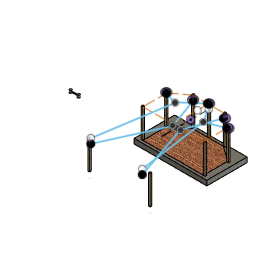
Mic Placements v4 (Autodesk Fusion 360 design; units mm, degrees)
Autodesk Fusion 360 part; units mm, degrees
sketch "Sketch1" plane through (0, 0, 0) normal (0, 1, 0) x (1, 0, 0)
  line L0 (0, 1104.9) -> (0, -342.9) construction
  line L1 (-1905, 1104.9) -> (1905, 1104.9) construction
  line L2 (-1905, -1104.9) -> (1905, -1104.9)
  line L3 (1905, -1104.9) -> (-1905, 1104.9) construction
  line L4 (-1905, -1104.9) -> (-1905, 1104.9) construction
  line L5 (0, -342.9) -> (0, 419.1) construction
  line L6 (0, 1104.9) -> (0, -342.9) construction
  line L7 (-1905, 419.1) -> (-952.5, 1104.9)
  line L8 (-1905, -342.9) -> (-1905, 1104.9) construction
  line L9 (-1905, 419.1) -> (-1905, -1104.9)
  line L10 (1905, 1104.9) -> (1905, -1104.9) construction
  line L11 (-1905, 1104.9) -> (0, 1104.9) construction
  line L12 (1905, -342.9) -> (1905, 1104.9) construction
  line L13 (1905, -342.9) -> (1905, 419.1) construction
  line L14 (0, -342.9) -> (1905, -342.9) construction
  line L15 (1905, 1104.9) -> (0, 1104.9) construction
  line L16 (1905, 419.1) -> (952.5, 1104.9) construction
  line L17 (-952.5, 1104.9) -> (952.5, 1104.9)
  line L18 (0, 1104.9) -> (0, -342.9) construction
  line L19 (1905, 419.1) -> (-1905, 419.1)
  line L20 (1905, -1104.9) -> (1905, 419.1)
  line L21 (-1905, -1104.9) -> (1905, 1104.9) construction
  line L22 (1905, -1104.9) -> (-1905, -1104.9) construction
  line L23 (0, -342.9) -> (-1905, -342.9) construction
  line L24 (1905, 419.1) -> (952.5, 1104.9)
  line L25 (1905, 419.1) -> (0, 419.1) construction
  line L26 (50.7492, 1206.3984) -> (50.7492, 1104.9)
  line L27 (952.5, 1104.9) -> (-952.5, 1104.9)
  line L28 (-1905, -1104.9) -> (1905, -1104.9)
  line L29 (-1905, -1104.9) -> (-2006.4984, -1104.9)
  line L30 (-2006.4984, 368.3508) -> (-2006.4984, 469.8492)
  line L31 (-1905, -1003.4016) -> (-1905, -1104.9)
  line L32 (952.5, 1104.9) -> (1054.1, 1104.9)
  line L33 (1054.1, 1206.5) -> (952.5, 1206.5)
  line L34 (1905, 419.1) -> (952.5, 1104.9)
  line L35 (0, 1104.9) -> (0, -1104.9) construction
  line L36 (1905, -1104.9) -> (2006.4984, -1104.9)
  line L37 (-1905, 368.3508) -> (-2006.4984, 469.8492) construction
  line L38 (-952.5, 1206.5) -> (-952.5, 1104.9)
  line L39 (50.7492, 1104.9) -> (-50.7492, 1206.3984) construction
  line L40 (-1905, 419.1) -> (-1955.7492, 419.1) construction
  line L41 (2006.4984, 368.3508) -> (1905, 469.8492) construction
  line L42 (0, 1104.9) -> (0, 1155.6492) construction
  line L43 (-1905, 419.1) -> (-1905, -1104.9)
  line L44 (-50.7492, 1104.9) -> (50.7492, 1206.3984) construction
  line L45 (-2006.4984, 469.8492) -> (-1905, 469.8492)
  line L46 (-50.7492, 1206.3984) -> (50.7492, 1206.3984)
  line L47 (-2006.4984, -1104.9) -> (-2006.4984, -1003.4016)
  line L48 (1905, -1003.4016) -> (1905, -1104.9)
  line L49 (-952.5, 1104.9) -> (-1905, 419.1)
  line L50 (-50.7492, 1104.9) -> (-50.7492, 1206.3984)
  line L51 (2006.4984, -1003.4016) -> (1905, -1003.4016)
  line L52 (-2006.4984, -1003.4016) -> (-1905, -1003.4016)
  line L53 (50.7492, 1104.9) -> (-50.7492, 1104.9)
  line L54 (1054.1, 1104.9) -> (1054.1, 1206.5)
  line L55 (-1905, 368.3508) -> (-2006.4984, 368.3508)
  line L56 (-1054.1, 1206.5) -> (-952.5, 1206.5)
  line L57 (2006.4984, -1104.9) -> (2006.4984, -1003.4016)
  line L58 (1905, 368.3508) -> (2006.4984, 469.8492) construction
  line L59 (-1054.1, 1104.9) -> (-1054.1, 1206.5)
  line L60 (1905, 419.1) -> (1955.7492, 419.1) construction
  line L61 (-1905, 469.8492) -> (-1905, 368.3508)
  line L62 (2006.4984, 469.8492) -> (1905, 469.8492)
  line L63 (1905, 469.8492) -> (1905, 368.3508)
  line L64 (-2006.4984, 368.3508) -> (-1905, 469.8492) construction
  line L65 (1905, 368.3508) -> (2006.4984, 368.3508)
  line L66 (-952.5, 1104.9) -> (-1054.1, 1104.9)
  line L67 (2006.4984, 368.3508) -> (2006.4984, 469.8492)
  line L68 (952.5, 1206.5) -> (952.5, 1104.9)
  line L69 (1905, -1104.9) -> (1905, 419.1)
  line L70 (2286, -1270) -> (-2286, -1270)
  line L71 (-2286, -1270) -> (-2286, 1270)
  line L72 (-2286, 1270) -> (2286, 1270)
  line L73 (2286, 1270) -> (2286, -1270)
  line L74 (2286, -1270) -> (-2286, 1270) construction
  line L75 (-2286, -1270) -> (2286, 1270) construction
  point P0 (-1955.7492, 419.1)
  point P1 (0, 1155.6492)
  point P2 (952.5, 1104.9)
  point P3 (1905, 419.1)
  point P4 (1905, -1104.9)
  point P5 (1955.7492, 419.1)
  dimension "d1" = 3810
  dimension "d2" = 2209.8
  dimension "d3" = 1447.8
  dimension "d4" = 762
  dimension "d5" = 762
  dimension "d8" = 101.6
  dimension "d9" = 101.6
  dimension "d10" = 50.7492
  dimension "d11" = 101.4984
  dimension "d12" = 101.4984
  dimension "d13" = 50.7492
  dimension "d14" = 101.4984
  dimension "d15" = 101.4984
  dimension "d16" = 101.4984
  dimension "d17" = 101.4984
  constraint horizontal L22
  constraint perpendicular L4 L22
  constraint parallel L1 L22
  constraint parallel L4 L10
  constraint coincident origin L3
  constraint coincident origin L21
  constraint midpoint L0.start L1
  constraint perpendicular L0 L1
  constraint horizontal L11
  constraint vertical L6
  constraint horizontal L23
  constraint vertical L8
  constraint horizontal L15
  constraint vertical L18
  constraint horizontal L14
  constraint vertical L12
  constraint perpendicular L5 L23
  constraint perpendicular L13 L14
  constraint midpoint P2 L15
  constraint horizontal L19
  constraint vertical L9
  constraint horizontal L2
  constraint vertical L20
  constraint midpoint L7.end L11
  constraint coincident L7.end L17.start
  constraint coincident L7.start L9.start
  constraint perpendicular L40 L43
  constraint perpendicular L30 L55
  constraint parallel L45 L55
  constraint parallel L30 L61
  constraint coincident P0 L37
  constraint coincident P0 L64
  constraint coincident P0 L40.end
  constraint midpoint L0.start L27
  constraint perpendicular L27 L42
  constraint perpendicular L50 L53
  constraint parallel L46 L53
  constraint parallel L26 L50
  constraint coincident P1 L39
  constraint coincident P1 L44
  constraint coincident P1 L42.end
  constraint coincident L2.start L4.start
  constraint midpoint L35.end L28
  constraint symmetric L7.start P3 L35
  constraint symmetric L2.start P4 L35
  constraint symmetric L7.end P2 L35
  constraint symmetric L59.start L32.end L35
  constraint symmetric L56.start L33.start L35
  constraint symmetric L38.start L33.end L35
  constraint symmetric P0 P5 L35
  constraint symmetric L37.start L58.start L35
  constraint symmetric L30.start L41.start L35
  constraint symmetric L30.end L58.end L35
  constraint symmetric L45.end L41.end L35
  constraint symmetric L29.end L36.end L35
  constraint symmetric L47.end L51.start L35
  constraint symmetric L48.start L31.start L35
  constraint horizontal L70
  constraint perpendicular L70 L71
  constraint parallel L70 L72
  constraint parallel L71 L73
  constraint coincident L74 origin
  constraint coincident L75 origin
  measures "d1" distance of L1.start L1.end
  measures "d2" distance of L2.start L1.start
  measures "d3" distance of L0.end L0.start
  measures "d4" distance of L0.end L5.end
  measures "d5" distance of L12.start P3
  measures "d8" distance of L59.start L7.end
  measures "d9" distance of L7.end L38.start
  measures "d10" distance of L7.start P0
  measures "d11" distance of L45.end L30.end
  measures "d12" distance of L30.start L30.end
  measures "d13" distance of L0.start P1
  measures "d14" distance of L39.end L26.start
  measures "d15" distance of L44.start L39.end
  measures "d16" distance of L2.start L29.end
  measures "d17" distance of L2.start L31.start
extrude "Extrude1" add sketch "Sketch1" along normal blind 1828.8 contours L9 L29 L31 L43 L47 L52 | L38 L56 L59 L66 | L32 L33 L54 L68 | L20 L36 L48 L51 L57 L69 | L9 L30 L43 L45 L55 L61 | L20 L62 L63 L65 L67 L69 | L17 L26 L27 L46 L50 L53 makes body 1 at (952.5, 609.6, -1172.6333) makes body 2 at (-986.3667, 609.6, -1104.9) makes body 3 at (-50.7492, 609.6, -1138.7328) makes body 4 at (1972.6656, 609.6, -469.8492) makes body 5 at (-1938.8328, 609.6, -368.3508) makes body 6 at (-1938.8328, 609.6, 1104.9) makes body 7 at (1905, 1219.2, 1071.0672)
extrude "Extrude2" add sketch "Sketch1" against normal blind 304.8 separate body makes body 8
extrude "Extrude3" add sketch "Sketch1" against normal blind 381 separate body contours L2 L9 L19 L20 L28 L31 L43 L48 L61 L63 L69 | L7 L17 L19 L24 L27 L34 L49 L53 makes body 9
ref_plane "WorkPlane1" through (0, 1828.8, 0) normal (0, 1, 0) x (0, 0, 1)
sketch "Sketch3" plane through (0, 1828.8, 0) normal (0, 1, 0) x (1, 0, 0)
  line L0 (-1905, 419.1) -> (-1905, -1104.9) construction
  line L1 (0, 1104.9) -> (0, -1104.9) construction
  line L2 (1905, -1104.9) -> (1905, 419.1) construction
  line L3 (952.5, 1104.9) -> (-952.5, 1104.9) construction
  line L4 (-1115.3442, 97.5223) -> (-1828.8, -4457.6999)
  line L5 (-1905, -1104.9) -> (1905, -1104.9) construction
  line L6 (831.349, -64.1091) -> (1469.5957, -4515.3092)
  line L7 (1905, 419.1) -> (952.5, 1104.9) construction
  line L8 (-952.5, 1104.9) -> (-1905, 419.1) construction
  line L9 (50.7492, 1104.9) -> (50.7492, 1206.3984)
  line L10 (50.7492, 1206.3984) -> (-50.7492, 1206.3984)
  line L11 (-50.7492, 1206.3984) -> (-50.7492, 1104.9)
  line L12 (-50.7492, 1104.9) -> (50.7492, 1104.9)
  line L13 (-1905, 469.8492) -> (-2006.4984, 469.8492)
  line L14 (-2006.4984, 469.8492) -> (-2006.4984, 368.3508)
  line L15 (-2006.4984, 368.3508) -> (-1905, 368.3508)
  line L16 (-1905, 368.3508) -> (-1905, 469.8492)
  line L17 (1905, 368.3508) -> (2006.4984, 368.3508)
  line L18 (2006.4984, 368.3508) -> (2006.4984, 469.8492)
  line L19 (2006.4984, 469.8492) -> (1905, 469.8492)
  line L20 (1905, 469.8492) -> (1905, 368.3508)
  line L21 (831.349, -64.1091) -> (820.5335, 11.3194) construction
  circle A0 centre (825.9413, -26.3949) radius 38.1
  line L22 (-1115.3442, 97.5223) -> (-1115.3442, 173.7223) construction
  circle A1 centre (-1115.3442, 135.6223) radius 38.1
  line L23 (-1153.3891, 137.6712) -> (-1905, 368.3508)
  line L24 (-1115.3442, 173.7223) -> (-50.7492, 1104.9)
  line L25 (812.5209, 9.2633) -> (50.7492, 1104.9)
  line L26 (788.4457, -33.1542) -> (1905, 368.3508)
  point P0 (0, 419.1)
  dimension "d37" = 76.2
  dimension "d38" = 76.2
  constraint midpoint L1.start L3
  constraint midpoint L1.end L5
  constraint parallel L6 L21
  constraint midpoint L21 A0.centre
  constraint coincident L21.end A0
  constraint vertical L22
  constraint midpoint L22 A1.centre
  constraint coincident L4.start A1
  constraint coincident A1 L23.start
  constraint coincident L15.end L16.start
  constraint coincident L11.end L12.start
  constraint coincident A0 L25.start
  constraint coincident L9.start L12.end
  constraint coincident A0 L26.start
  constraint coincident L17.start L20.end
  measures "d37" distance of L6.start L21.end
  measures "d38" distance of L4.start L22.end
ref_plane "WorkPlane3" through (0, 1524, 0) normal (0, 1, 0) x (0, 0, 1)
sketch "Sketch4" plane through (0, 1524, 0) normal (0, 1, 0) x (1, 0, 0)
  line L0 (0, 1143) -> (0, -1778) construction
  line L1 (0, -1778) -> (0, 0) construction
  line L2 (175, -876.3) -> (-175, -876.3)
  line L3 (-175, -876.3) -> (-175, -901.7)
  line L4 (-175, -901.7) -> (175, -901.7)
  line L5 (175, -901.7) -> (175, -876.3)
  line L6 (175, -876.3) -> (-175, -901.7) construction
  line L7 (-175, -876.3) -> (175, -901.7) construction
  line L8 (-175, -889) -> (-251.2, -889) construction
  line L9 (175, -889) -> (251.2, -889) construction
  circle A0 centre (251.2, -889) radius 76.2
  circle A1 centre (-251.2, -889) radius 76.2
  line L10 (-1828.8, -4457.6999) -> (-256.5809, -965.0098)
  line L11 (-952.5, 1104.9) -> (-952.5, 1206.5)
  line L12 (-952.5, 1206.5) -> (-1054.1, 1206.5)
  line L13 (-1054.1, 1206.5) -> (-1054.1, 1104.9)
  line L14 (-1054.1, 1104.9) -> (-952.5, 1104.9)
  line L15 (952.5, 1206.5) -> (952.5, 1104.9)
  line L16 (952.5, 1104.9) -> (1054.1, 1104.9)
  line L17 (1054.1, 1104.9) -> (1054.1, 1206.5)
  line L18 (1054.1, 1206.5) -> (952.5, 1206.5)
  line L19 (-256.5809, -965.0098) -> (-256.5809, -812.9902) construction
  line L20 (255.2053, -965.0946) -> (255.2053, -812.9053) construction
  line L21 (-952.5, 1104.9) -> (-256.5809, -812.9902)
  line L22 (952.5, 1104.9) -> (255.2053, -812.9053)
  line L23 (255.2053, -965.0946) -> (1469.5957, -4515.3092)
  line L24 (-175, -901.7) -> (-176.0658, -901.7)
  line L25 (-175, -876.3) -> (-176.0658, -876.3)
  line L26 (175, -876.3) -> (176.0658, -876.3)
  line L27 (175, -901.7) -> (176.0658, -901.7)
  point P0 (0, -889)
  point P1 (-1828.8, -4457.6999)
  point P2 (1469.5957, -4515.3092)
  dimension "d27" = 350
  dimension "d28" = 25.4
  dimension "d29" = 76.2
  dimension "d30" = 76.2
  constraint vertical L0
  constraint coincident L1.end origin
  constraint parallel L0 L1
  constraint horizontal L2
  constraint perpendicular L2 L3
  constraint parallel L2 L4
  constraint parallel L3 L5
  constraint coincident L6 P0
  constraint coincident L7 P0
  constraint midpoint L1 P0
  constraint midpoint L3 L8.start
  constraint perpendicular L3 L8
  constraint midpoint L5 L9.start
  constraint perpendicular L5 L9
  constraint coincident L9.end A0.centre
  constraint coincident L9.start A0
  constraint coincident L8.end A1.centre
  constraint coincident L8.start A1
  constraint coincident P1 L10.start
  constraint coincident A1 L10.end
  constraint coincident A1 L19.end
  constraint perpendicular L8 L19
  constraint coincident A0 L20.start
  constraint coincident A0 L20.end
  constraint perpendicular L4 L20
  constraint coincident L11.start L14.end
  constraint coincident L15.end L16.start
  constraint coincident P2 L23.end
  constraint coincident A1 L24.end
  constraint perpendicular L3 L24
  constraint coincident A1 L25.end
  constraint perpendicular L3 L25
  constraint coincident A0 L26.end
  constraint perpendicular L5 L26
  constraint coincident A0 L27.end
  constraint perpendicular L5 L27
  measures "d27" distance of L3.end L4.end
  measures "d28" distance of L2.end L3.end
  measures "d29" distance of L8.start L8.end
  measures "d30" distance of L9.start L9.end
sketch "Sketch5" plane through (0, 0, 0) normal (0, 1, 0) x (-1, 0, 0)
  line L0 (-1054.1, -1104.9) -> (-952.5, -1104.9)
  line L1 (-952.5, -1104.9) -> (-1905, -419.1)
  line L2 (-1905, -419.1) -> (-1905, -469.8492)
  line L3 (-1905, -469.8492) -> (-2006.4984, -469.8492)
  line L4 (-2006.4984, -469.8492) -> (-2006.4984, -368.3508)
  line L5 (-2006.4984, -368.3508) -> (-1905, -368.3508)
  line L6 (-1905, -368.3508) -> (-1905, 1003.4016)
  line L7 (-1905, 1003.4016) -> (-2006.4984, 1003.4016)
  line L8 (-2006.4984, 1003.4016) -> (-2006.4984, 1104.9)
  line L9 (-2006.4984, 1104.9) -> (2006.4984, 1104.9)
  line L10 (2006.4984, 1104.9) -> (2006.4984, 1003.4016)
  line L11 (2006.4984, 1003.4016) -> (1905, 1003.4016)
  line L12 (1905, 1003.4016) -> (1905, -368.3508)
  line L13 (1905, -368.3508) -> (2006.4984, -368.3508)
  line L14 (2006.4984, -368.3508) -> (2006.4984, -469.8492)
  line L15 (2006.4984, -469.8492) -> (1905, -469.8492)
  line L16 (1905, -469.8492) -> (1905, -419.1)
  line L17 (1905, -419.1) -> (952.5, -1104.9)
  line L18 (952.5, -1104.9) -> (1054.1, -1104.9)
  line L19 (1054.1, -1104.9) -> (1054.1, -1206.5)
  line L20 (1054.1, -1206.5) -> (952.5, -1206.5)
  line L21 (952.5, -1206.5) -> (952.5, -1104.9)
  line L22 (952.5, -1104.9) -> (50.7492, -1104.9)
  line L23 (50.7492, -1104.9) -> (50.7492, -1206.3984)
  line L24 (50.7492, -1206.3984) -> (-50.7492, -1206.3984)
  line L25 (-50.7492, -1206.3984) -> (-50.7492, -1104.9)
  line L26 (-50.7492, -1104.9) -> (-952.5, -1104.9)
  line L27 (-952.5, -1104.9) -> (-952.5, -1206.5)
  line L28 (-952.5, -1206.5) -> (-1054.1, -1206.5)
  line L29 (-1054.1, -1206.5) -> (-1054.1, -1104.9)
  line L30 (-2286, -1270) -> (2286, -1270)
  line L31 (2286, -1270) -> (2286, 1270)
  line L32 (2286, 1270) -> (-2286, 1270)
  line L33 (-2286, 1270) -> (-2286, -1270)
  line L34 (1905, 1104.9) -> (1905, 4457.6999) construction
  line L35 (-1905, 1104.9) -> (-1905, 4457.6999) construction
  line L36 (-1905, 4457.6999) -> (1905, 4457.6999) construction
  line L37 (1854.2, 4508.4999) -> (1955.8, 4508.4999)
  line L38 (1955.8, 4508.4999) -> (1955.8, 4406.8999)
  line L39 (1955.8, 4406.8999) -> (1854.2, 4406.8999)
  line L40 (1854.2, 4406.8999) -> (1854.2, 4508.4999)
  line L41 (1854.2, 4508.4999) -> (1955.8, 4406.8999) construction
  line L42 (1955.8, 4508.4999) -> (1854.2, 4406.8999) construction
  line L43 (-1955.8, 4508.4999) -> (-1854.2, 4508.4999)
  line L44 (-1854.2, 4508.4999) -> (-1854.2, 4406.8999)
  line L45 (-1854.2, 4406.8999) -> (-1955.8, 4406.8999)
  line L46 (-1955.8, 4406.8999) -> (-1955.8, 4508.4999)
  line L47 (-1955.8, 4508.4999) -> (-1854.2, 4406.8999) construction
  line L48 (-1854.2, 4508.4999) -> (-1955.8, 4406.8999) construction
  point P0 (1828.8, 4457.6999)
  point P1 (-1469.5957, 4515.3092)
  point P2 (1905, 4457.6999)
  point P3 (-1905, 4457.6999)
  dimension "d31" = 101.6
  dimension "d32" = 101.6
  dimension "d33" = 101.6
  dimension "d34" = 101.6
  constraint coincident L9 L34.start
  constraint perpendicular L32 L34
  constraint coincident L9 L35.start
  constraint perpendicular L32 L35
  constraint perpendicular L34 L36
  constraint horizontal L37
  constraint perpendicular L37 L38
  constraint parallel L37 L39
  constraint parallel L38 L40
  constraint coincident L41 P2
  constraint coincident L42 P2
  constraint coincident P2 L34.end
  constraint horizontal L43
  constraint perpendicular L43 L44
  constraint parallel L43 L45
  constraint parallel L44 L46
  constraint coincident L47 P3
  constraint coincident L48 P3
  constraint coincident P3 L35.end
  measures "d31" distance of L38.end L39.end
  measures "d32" distance of L37.end L38.end
  measures "d33" distance of L44.end L45.end
  measures "d34" distance of L43.end L44.end
extrude "Extrude4" add sketch "Sketch5" along normal blind 1828.8 separate body contours L37 L38 L39 L40 | L43 L44 L45 L46 makes body 10 at (-1888.0667, 609.6, 4508.4999) makes body 11 at (1921.9333, 609.6, 4508.4999)
sketch "Sketch6" plane through (0, 0, 0) normal (0, 1, 0) x (1, 0, 0)
  line L0 (-6779, -705.2707) -> (-6780.0658, -705.2707)
  line L1 (-6429, -679.8707) -> (-6427.9342, -679.8707)
  line L2 (-6779, -679.8707) -> (-6429, -705.2707) construction
  circle A0 centre (-6855.2, -692.5707) radius 76.2
  line L3 (-6779, -705.2707) -> (-6429, -705.2707)
  line L4 (-6855.2, -768.7707) -> (-6855.2, -616.3707) construction
  circle A1 centre (-6352.8, -692.5707) radius 76.2
  line L5 (-6779, -679.8707) -> (-6780.0658, -679.8707)
  line L6 (-6429, -705.2707) -> (-6427.9342, -705.2707)
  line L7 (-6429, -705.2707) -> (-6429, -679.8707)
  line L8 (-6352.8, -768.7707) -> (-6352.8, -616.3707) construction
  line L9 (-6779, -692.5707) -> (-6855.2, -692.5707) construction
  line L10 (-6429, -679.8707) -> (-6779, -679.8707)
  line L11 (-6429, -692.5707) -> (-6352.8, -692.5707) construction
  line L12 (-6779, -679.8707) -> (-6779, -705.2707)
  line L13 (-6429, -679.8707) -> (-6779, -705.2707) construction
  point P0 (-6604, -692.5707)
  dimension "d39" = 350
  dimension "d40" = 25.4
  dimension "d41" = 76.2
  dimension "d42" = 76.2
  constraint horizontal L10
  constraint perpendicular L10 L12
  constraint parallel L3 L10
  constraint parallel L7 L12
  constraint coincident P0 L13
  constraint coincident P0 L2
  constraint midpoint L9.start L12
  constraint perpendicular L9 L12
  constraint midpoint L11.start L7
  constraint perpendicular L7 L11
  constraint coincident A1.centre L11.end
  constraint coincident L11.start A1
  constraint coincident A0.centre L9.end
  constraint coincident L9.start A0
  constraint coincident L4.start A0
  constraint coincident L4.end A0
  constraint perpendicular L4 L9
  constraint coincident L8.start A1
  constraint coincident L8.end A1
  constraint perpendicular L3 L8
  constraint coincident L0.end A0
  constraint perpendicular L0 L12
  constraint coincident L5.end A0
  constraint perpendicular L5 L12
  constraint coincident L1.end A1
  constraint perpendicular L1 L7
  constraint coincident L6.end A1
  constraint perpendicular L6 L7
  measures "d39" distance of L0.start L2.end
  measures "d40" distance of L0.start L2.start
  measures "d41" distance of L9.start A0.centre
  measures "d42" distance of L11.start A1.centre
extrude "Extrude5" add sketch "Sketch6" along normal mid plane 152.4 separate body contours A0 | A1 makes body 12 at (-6868.432, -25.4, 767.6131) makes body 13 at (-6331.4073, 76.2, 674.1041)
extrude "Extrude6" add sketch "Sketch6" along normal mid plane 50.8 contours L3 L7 L10 L12 | L0 A0 L12 | A1 L6 L7 | A0 L5 L12 | L1 A1 L7 bodies 12 13
